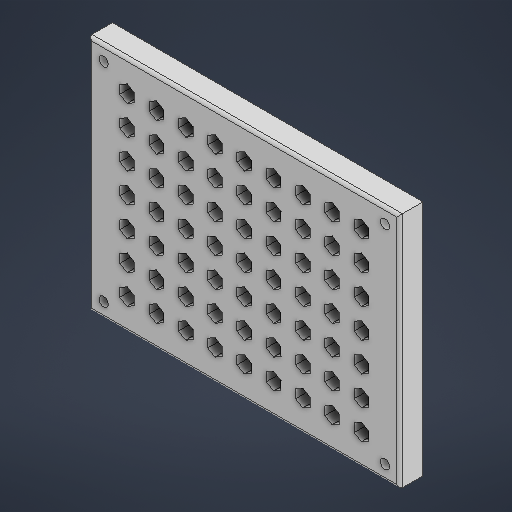
# Autodesk Inventor part: air-monitor_lid
Saved by Autodesk Inventor 2026.1 (Build 301233020, 233B)
## iProperties
Created: 2026-06-10
Part Number: air-monitor_lid
Material: Generic
Document SubType Name: Modeling
Designer: astro
Density: 1 g/cm^3
Appearance: Default
Author: astro
Autodesk Inventor part; units mm, degrees
ref_plane "YZ Plane" through (0, 0, 0) normal (1, 0, 0) x (0, 1, 0)
ref_plane "XZ Plane" through (0, 0, 0) normal (0, 1, 0) x (-1, 0, 0)
ref_plane "XY Plane" through (0, 0, 0) normal (0, 0, 1) x (1, 0, 0)
sketch "Sketch1" plane through (0, 0, 0) normal (0, 0, 1) x (1, 0, 0)
  line L0 (0, 0) -> (106, 0)
  line L1 (106, 0) -> (106, 81)
  line L2 (106, 81) -> (0, 81)
  line L3 (0, 81) -> (0, 0)
  dimension "d0" = 106
  dimension "d1" = 81
  constraints: 8 end point, 2 parallel, 1 horizontal, 1 perpendicular
  measures "d0" distance of L2.end L1.end
  measures "d1" distance of L1.end L0.end
extrude "Extrusion1" add sketch "Sketch1" along normal blind 5
sketch "Sketch2" plane through (0, 0, 0) normal (0, 0, -1) x (-1, 0, 0)
  line L0 (-1.5, 79.5) -> (-104.5, 79.5)
  line L1 (-104.5, 79.5) -> (-104.5, 1.5)
  line L2 (-104.5, 1.5) -> (-1.5, 1.5)
  line L3 (-1.5, 1.5) -> (-1.5, 79.5)
  line L4 (-106, 81) -> (0, 81)
  line L5 (0, 81) -> (0, 0)
  line L6 (0, 0) -> (-106, 0)
  line L7 (-106, 0) -> (-106, 81)
  constraints: 16 end point, 4 parallel, 2 perpendicular, 1 horizontal
extrude "Extrusion2" add sketch "Sketch2" along normal blind 3
sketch "Sketch3" plane through (0, 0, 5) normal (0, 0, 1) x (1, 0, 0)
  line L0 (53, 43.39) -> (55.5028, 41.945)
  line L1 (55.5028, 41.945) -> (55.5028, 39.055)
  line L2 (55.5028, 39.055) -> (53, 37.61)
  line L3 (53, 37.61) -> (50.4972, 39.055)
  line L4 (50.4972, 39.055) -> (50.4972, 41.945)
  line L5 (50.4972, 41.945) -> (53, 43.39)
  line L6 (106, 81) -> (0, 81) projected
  line L7 (0, 81) -> (0, 0) projected
  point P0 (53, 40.5)
  dimension "d7" = 2.89
  dimension "d8" = 40.5
  dimension "d9" = 53
  constraints: 12 end point, 1 vertical, 13 other
  measures "d7" distance of L0.start point (53, 40.5)
  measures "d8" distance from line of L6 point (53, 40.5)
  measures "d9" distance from line of L7 point (53, 40.5)
extrude "Extrusion3" cut sketch "Sketch3" against normal blind 5
pattern_linear "Rectangular Pattern1" count 5 spacing 10 along (-1, 0, 0) count 4 spacing 10 along (0, -1, 0) of "Extrusion3"
pattern_linear "Rectangular Pattern2" count 5 spacing 10 along (1, 0, 0) count 4 spacing 10 along (0, -1, 0) of "Extrusion3"
pattern_linear "Rectangular Pattern3" count 5 spacing 10 along (-1, 0, 0) count 4 spacing 10 along (0, 1, 0) of "Extrusion3"
pattern_linear "Rectangular Pattern4" count 5 spacing 10 along (1, 0, 0) count 4 spacing 10 along (0, 1, 0) of "Extrusion3"
sketch "Sketch4" plane through (0, 0, 5) normal (0, 0, 1) x (1, 0, 0)
  circle A0 centre (5, 76) radius 1.6
  circle A1 centre (5, 5) radius 1.6
  circle A2 centre (101, 76) radius 1.6
  circle A3 centre (101, 5) radius 1.6
  line L0 (106, 81) -> (0, 81) projected
  line L1 (0, 81) -> (0, 0) projected
  line L2 (0, 0) -> (106, 0) projected
  line L3 (106, 0) -> (106, 81) projected
  dimension "d36" = 3.2
  dimension "d37" = 3.2
  dimension "d38" = 3.2
  dimension "d39" = 3.2
  dimension "d40" = 5
  dimension "d41" = 5
  dimension "d42" = 5
  dimension "d43" = 5
  dimension "d44" = 5
  dimension "d45" = 5
  dimension "d46" = 5
  dimension "d47" = 5
  constraints: 4 centre point
  measures "d36" diameter of A0
  measures "d37" diameter of A1
  measures "d38" diameter of A2
  measures "d39" diameter of A3
  measures "d40" distance from line of L0 A0.centre
  measures "d41" distance from line of L1 A0.centre
  measures "d42" distance from line of L1 A1.centre
  measures "d43" distance from line of L2 A1.centre
  measures "d44" distance from line of L3 A3.centre
  measures "d45" distance from line of L2 A3.centre
  measures "d46" distance from line of L0 A2.centre
  measures "d47" distance from line of L3 A2.centre
extrude "Extrusion4" cut sketch "Sketch4" against normal blind 5 contours A0 | A1 | A2 | A3
fillet "Fillet1" radius 1 4 edges at (0, 40.5, 5) (53, 81, 5) (106, 40.5, 5) (53, 0, 5)
body "Solid1"
